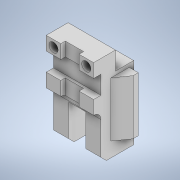
# Autodesk Inventor part: 2.8
Saved by Autodesk Inventor 2022 (Build 260153000, 153)
## iProperties
Created: 2023-04-17
Part Number: 2.8
Material: Genérico
Document SubType Name: Modeling
Designer: jpjoa
Density: 1 g/cm^3
Appearance: Padrão
Author: jpjoa
Autodesk Inventor part; units mm, degrees
ref_plane "YZ Plane" through (0, 0, 0) normal (1, 0, 0) x (0, 1, 0)
ref_plane "XZ Plane" through (0, 0, 0) normal (0, 1, 0) x (-1, 0, 0)
ref_plane "XY Plane" through (0, 0, 0) normal (0, 0, 1) x (1, 0, 0)
sketch "Esboço1" plane through (0, 0, 0) normal (0, 0, 1) x (1, 0, 0)
  line L0 (0, 0) -> (16.5, 0)
  line L1 (16.5, 0) -> (16.5, 41)
  line L2 (16.5, 41) -> (35.5, 41)
  line L3 (35.5, 41) -> (35.5, 0)
  line L4 (35.5, 0) -> (52, 0)
  line L5 (52, 0) -> (52, 50)
  line L6 (52, 50) -> (0, 50)
  line L7 (0, 50) -> (0, 0)
  line L8 (52, 50) -> (52, 65)
  line L9 (52, 65) -> (0, 65)
  line L10 (0, 65) -> (0, 50)
  line L11 (52, 65) -> (52, 85)
  line L12 (52, 85) -> (0, 85)
  line L13 (0, 85) -> (0, 65)
  line L14 (52, 85) -> (52, 100)
  line L15 (52, 100) -> (0, 100)
  line L16 (0, 100) -> (0, 85)
  circle A0 centre (8, 92.5) radius 5
  circle A1 centre (44, 92.5) radius 5
  line L17 (36, 100) -> (36, 85)
  line L18 (16, 100) -> (16, 85)
  line L19 (36, 50) -> (36, 65)
  line L20 (16, 65) -> (16, 50)
  line L21 (52, 80) -> (0, 80)
  point P0 (36, 92.5)
  point P1 (36, 57.5)
  point P2 (16, 92.5)
  point P3 (16, 57.5)
  dimension "d0" = 19
  dimension "d1" = 52
  dimension "d2" = 41
  dimension "d3" = 100
  dimension "d4" = 15
  dimension "d5" = 20
  dimension "d6" = 50
  dimension "d7" = 10
  dimension "d8" = 10
  dimension "d9" = 36
  dimension "d10" = 20
  dimension "d12" = 16
  dimension "d13" = 16
  dimension "d14" = 8
  dimension "d15" = 8
  dimension "d16" = 7.5
  dimension "d17" = 7.5
  dimension "d18" = 20
  constraints: 44 end point, 16 perpendicular, 14 point on line, 4 midpoint, 2 centre point, 2 horizontal, 2 vertical, 2 vertical alignment, 1 collinear
  measures "d0" distance of L3.end L0.end
  measures "d1" distance of L4.end L0.start
  measures "d2" distance between parallel lines of L0 L2
  measures "d3" distance of L15.end L0.start
  measures "d4" distance of L12.end L15.end
  measures "d5" distance between parallel lines of L9 L12
  measures "d6" distance between parallel lines of L6 L15
  measures "d7" diameter of A0
  measures "d8" diameter of A1
  measures "d9" distance of A1.centre A0.centre
  measures "d10" distance between parallel lines of L18 L17
  measures "d12" distance between parallel lines of L14 L17
  measures "d13" distance between parallel lines of L16 L18
  measures "d14" distance from line of L14 A1.centre
  measures "d15" distance from line of L16 A0.centre
  measures "d16" distance from line of L12 A1.centre
  measures "d17" distance from line of L15 A1.centre
  measures "d18" distance between parallel lines of L21 L15
extrude "Extrusão1" add sketch "Esboço1" along normal blind 24 contours L10 L9 L20 L6 | L19 L9 L8 L6 | L16 L15 L18 L12 | L12 L17 L15 L14
extrude "Extrusão2" add sketch "Esboço1" along normal blind 16 contours L7 L6 L5 L4 L3 L2 L1 L0 | L13 L21 L11 L9 | L13 L12 L11 L21
extrude "Extrusão3" add sketch "Esboço1" along normal blind 19 contours L20 L9 L19 L6 | L18 L15 L17 L12
extrude "Extrusão4" add sketch "Esboço1" against normal blind 20 contours L7 L6 L5 L4 L3 L2 L1 L0 | L10 L9 L20 L6 | L20 L9 L19 L6 | L13 L21 L11 L9 | L19 L9 L8 L6
chamfer "Chanfro1" distance 6 angle 45 2 edges at (8.25, 0, 16) (43.75, 0, 16)
fillet "Arredondamento1" radius 8 1 edges at (26, 50, 16)
sketch "Esboço2" plane through (52, 85, 24) normal (1, 0, 0) x (0, 0, -1)
  line L0 (39, -69) -> (39, -9)
  line L1 (39, -9) -> (19, -9)
  line L2 (19, -9) -> (19, -69)
  line L3 (19, -69) -> (39, -69)
  line L4 (44, -85) -> (14, -85) projected
  line L5 (44, -5) -> (44, -85) projected
  point P0 (24, -85)
  dimension "d31" = 60
  dimension "d32" = 20
  dimension "d34" = 16
  dimension "d35" = 5
  constraints: 8 end point, 2 perpendicular, 1 vertical
  measures "d31" distance of L0.start L0.end
  measures "d32" distance of L0.end L1.end
  measures "d34" distance between parallel lines of L4 L3
  measures "d35" distance between parallel lines of L5 L0
extrude "Extrusão5" add sketch "Esboço2" along normal blind 10
sketch "Esboço3" plane through (0, 85, 24) normal (-1, 0, 0) x (0, 0, 1)
  line L0 (-39, -9) -> (-39, -69)
  line L1 (-39, -69) -> (-19, -69)
  line L2 (-19, -69) -> (-19, -9)
  line L3 (-19, -9) -> (-39, -9)
  line L4 (-44, -85) -> (-14, -85) projected
  line L5 (-44, -85) -> (-44, -5) projected
  point P0 (-24, -85)
  dimension "d38" = 60
  dimension "d39" = 20
  dimension "d40" = 16
  dimension "d41" = 5
  constraints: 8 end point, 3 perpendicular, 1 vertical
  measures "d38" distance of L0.start L0.end
  measures "d39" distance between parallel lines of L0 L2
  measures "d40" distance between parallel lines of L4 L1
  measures "d41" distance between parallel lines of L5 L0
extrude "Extrusão6" add sketch "Esboço3" along normal blind 10
sketch "Esboço4" plane through (52, 16, -15) normal (0, -1, 0) x (1, 0, 0)
  line L0 (-52, 0) -> (-62, 0) projected
  line L1 (-62, 0) -> (-62, 20) projected
  line L2 (-52, -5) -> (-52, 25) projected
  line L3 (-62, 20) -> (-52, 20)
  line L4 (-52, -10.9123) -> (-52, 20)
  line L5 (-52, 20) -> (-70.0402, -5.7641)
  line L6 (-62, 20) -> (-70.0402, -5.7641)
  line L7 (0, 20) -> (10, 20) projected
  line L8 (18.4818, 20) -> (0, 20)
  line L9 (0, 20) -> (0, -16.4108)
  line L10 (0, 20) -> (27.6787, -19.5293)
  line L11 (18.4818, 20) -> (27.6787, -19.5293)
  point P0 (-52, 15)
  dimension "d46" = 35
  dimension "d47" = 35
  constraints: 16 end point, 2 collinear, 2 perpendicular, 2 point on line
  measures "d46" angle of L2 L5
  measures "d47" angle of L9 L10
extrude "Extrusão7" cut sketch "Esboço4" against normal through all contours L5 L1 L3 | L5 L6 L1 | L7 L8 L11 L10
equation "\"d14\" = d15"
equation "\"d16\" = d17"
